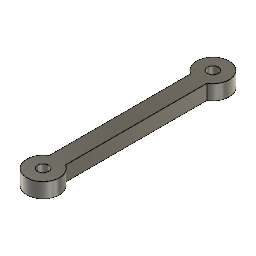
ensamble v16 (Autodesk Fusion 360 archive; units mm, degrees)
design "Eslabon esbelto"
Autodesk Fusion 360 part; units mm, degrees
sketch "Sketch1" plane through (0, 0, 0) normal (0, 1, 0) x (1, 0, 0)
sketch "Sketch2" plane through (0, 0, 0) normal (0, 0, 1) x (1, 0, 0)
  line L0 (-16.2522, 73.2678) -> (-16.2522, 11.1678)
  line L1 (-10.1922, 11.1678) -> (-10.1922, 73.2678)
  circle A0 centre (-13.2222, 73.2678) radius 2
  circle A1 centre (-13.2222, 73.2678) radius 6
  line L2 (-15.6922, 42.2178) -> (-4.6922, 42.2178)
  circle A2 centre (-13.2222, 11.1678) radius 2
  circle A3 centre (-13.2222, 11.1678) radius 6
  dimension "d1" = 6.06
  dimension "d2" = 62.1
  dimension "d3" = 4
  dimension "d4" = 12
  constraint vertical L0
  constraint vertical L1
  constraint concentric A0 A1
  constraint perpendicular L1 L2
  constraint midpoint L1 L2
  constraint symmetric A0 L2 A2
  constraint symmetric A1 L2 A3
  measures "d1" distance of L1.end L0.start
  measures "d2" distance of L1.end L1.start
  measures "d3" diameter of A0
  measures "d4" diameter of A1
extrude "Extrude1" add sketch "Sketch2" along normal blind 5.5
sketch "Sketch3" plane through (0, 0, 5.5) normal (0, 0, 1) x (-1, 0, 0)
  circle A0 centre (13.2222, -11.1678) radius 2
  circle A1 centre (13.2222, -73.2678) radius 2
  arc A2 (16.2522, -16.3465) -> (10.1922, -16.3465) centre (13.2222, -11.1678) ccw
  line L0 (10.1922, -16.3465) -> (10.1922, -68.0891)
  arc A3 (10.1922, -68.0891) -> (16.2522, -68.0891) centre (13.2222, -73.2678) ccw
  line L1 (16.2522, -68.0891) -> (16.2522, -16.3465)
  line L2 (13.2222, -16.3465) -> (21.0096, -16.3465)
  line L3 (21.0096, -16.3465) -> (21.0096, -5.1678)
  line L4 (21.0096, -5.1678) -> (13.2222, -5.1678)
  line L5 (13.2222, -5.1678) -> (13.2222, -16.3465)
  dimension "d10" = 62.1
  dimension "d11" = 68.1
  constraint horizontal L2
  constraint vertical L3
  constraint horizontal L4
  constraint vertical L5
  measures "d10" distance of A0.centre A1.centre
  measures "d11" distance of A1.centre L4

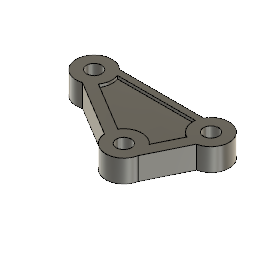
design "triangulo"
Autodesk Fusion 360 part; units mm, degrees
sketch "Sketch1" plane through (0, 0, 0) normal (0, 0, 1) x (1, 0, 0)
  line L0 (3.6773, 16.0313) -> (22.0441, 4.9587)
  line L1 (33.9267, 4.3237) -> (40.3034, 17.2878)
  line L2 (33.9155, 26.0059) -> (6.063, 26.0059)
  circle A0 centre (1.8404, 21.7433) radius 2.5
  circle A1 centre (39.2125, 23.1878) radius 2.5
  circle A2 centre (28.0267, 5.4148) radius 2.5
  circle A3 centre (1.8404, 21.7433) radius 6
  circle A4 centre (39.2125, 23.1878) radius 6
  circle A5 centre (28.0267, 5.4148) radius 6
  line L3 (7.4371, 23.9059) -> (33.2557, 23.9059)
  line L4 (6.7359, 18.2742) -> (22.8989, 8.5302)
  line L5 (32.5192, 9.392) -> (36.639, 17.7677)
  dimension "d6" = 5
  dimension "d7" = 12
  dimension "d8" = 12
  dimension "d9" = 12
  dimension "d10" = 2.1
  dimension "d12" = 3.5
  dimension "d13" = 3.5
  dimension "d23" = 21
  dimension "d25" = 37.4
  dimension "d26" = 30.86
  constraint horizontal L2
  constraint equal A0 A1
  constraint equal A0 A2
  constraint concentric A1 A4
  constraint concentric A2 A5
  constraint concentric A0 A3
  constraint coincident A3 L3.start
  constraint coincident A4 L3.end
  constraint parallel L2 L3
  constraint coincident A3 L4.start
  constraint coincident A5 L4.end
  constraint parallel L0 L4
  constraint coincident A5 L5.start
  constraint coincident A4 L5.end
  constraint parallel L1 L5
  constraint coincident L2.end A3
  constraint coincident L2.start A4
  constraint coincident L1.end A4
  constraint coincident L1.start A5
  constraint coincident L0.start A3
  constraint coincident L0.end A5
  measures "d6" diameter of A0
  measures "d7" diameter of A3
  measures "d8" diameter of A4
  measures "d9" diameter of A5
  measures "d10" distance of L2 L3
  measures "d12" distance of L0 L4
  measures "d13" distance of L1 L5
  measures "d23" distance of A1.centre A2.centre
  measures "d25" distance of A0.centre A1.centre
  measures "d26" distance of A0.centre A2.centre
extrude "Extrude1" add sketch "Sketch1" along normal blind 4 contours L0 A3 A5 L4 | A3 | A5 | L2 A3 A4 L3 | A3 A4 A5 L3 L4 L5 | A4
extrude "Extrude2" add sketch "Sketch1" along normal blind 7 and the other way blind 0.5 contours L0 A3 A5 L4 | A3 | A5 | L2 A3 A4 L3 | L1 A4 A5 L5 | A4
extrude "Extrude4" add 1 faces at (22.1509, 18.7206, 4) along direction (0, 0, 1) blind 2
sketch "Sketch2" plane through (0, 0, 7) normal (0, 0, 1) x (-1, 0, 0)
  circle A0 centre (-39.2125, -23.1878) radius 2.5
  circle A1 centre (-1.8404, -21.7433) radius 2.5
  circle A2 centre (-28.0267, -5.4148) radius 2.5
  line L0 (-3.6773, -16.0313) -> (-22.0441, -4.9587)
  arc A3 (-22.0441, -4.9587) -> (-33.9267, -4.3237) centre (-28.0267, -5.4148) ccw
  line L1 (-33.9267, -4.3237) -> (-40.3034, -17.2878)
  arc A4 (-40.3034, -17.2878) -> (-33.9155, -26.0059) centre (-39.2125, -23.1878) ccw
  line L2 (-33.9155, -26.0059) -> (-6.063, -26.0059)
  arc A5 (-6.063, -26.0059) -> (-3.6773, -16.0313) centre (-1.8404, -21.7433) ccw
sketch "Sketch3" plane through (0, 0, -0.5) normal (0, 0, -1) x (1, 0, 0)
  circle A0 centre (39.2125, -23.1878) radius 2.5
  circle A1 centre (1.8404, -21.7433) radius 2.5
  circle A2 centre (28.0267, -5.4148) radius 2.5
  line L0 (6.7359, -18.2742) -> (22.8989, -8.5302)
  arc A3 (22.8989, -8.5302) -> (32.5192, -9.392) centre (28.0267, -5.4148) ccw
  line L1 (32.5192, -9.392) -> (36.639, -17.7677)
  arc A4 (36.639, -17.7677) -> (33.2557, -23.9059) centre (39.2125, -23.1878) ccw
  line L2 (33.2557, -23.9059) -> (7.4371, -23.9059)
  arc A5 (7.4371, -23.9059) -> (6.7359, -18.2742) centre (1.8404, -21.7433) ccw
  line L3 (22.0441, -4.9587) -> (3.6773, -16.0313)
  arc A6 (3.6773, -16.0313) -> (6.063, -26.0059) centre (1.8404, -21.7433) ccw
  line L4 (6.063, -26.0059) -> (33.9155, -26.0059)
  arc A7 (33.9155, -26.0059) -> (40.3034, -17.2878) centre (39.2125, -23.1878) ccw
  line L5 (40.3034, -17.2878) -> (33.9267, -4.3237)
  arc A8 (33.9267, -4.3237) -> (22.0441, -4.9587) centre (28.0267, -5.4148) ccw
  line L6 (-4.1596, -29.1878) -> (45.2125, -29.1878)
  line L7 (45.2125, -29.1878) -> (45.2125, 0.5852)
  line L8 (45.2125, 0.5852) -> (-4.1596, 0.5852)
  line L9 (-4.1596, 0.5852) -> (-4.1596, -29.1878)
  dimension "d29" = 49.3721
  dimension "d30" = 29.773
  constraint horizontal L6
  constraint vertical L7
  constraint horizontal L8
  constraint vertical L9
  constraint tangent A7 L7
  constraint tangent A6 L9
  constraint tangent A8 L8
  constraint tangent A7 L6
  measures "d29" distance of L7.end L8.end
  measures "d30" distance of L6.start L8.end
equation "d_triang_ext = 16 mm"
equation "d_hueco_m4 = 5 mm"
equation "d6 = d_hueco_m4"
equation "l_borde_tri = 4 mm"
equation "d23 = 16 mm + 5 mm"
equation "d25 = 32.4 mm + 5 mm"
equation "d26 = 25.86 mm + 5 mm"

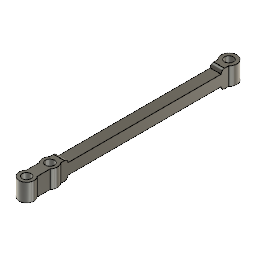
design "Barra marco"
Autodesk Fusion 360 part; units mm, degrees
sketch "Sketch1" plane through (0, 0, 0) normal (0, 0, 1) x (1, 0, 0)
  line L0 (-5, 83.0364) -> (1.2, 83.0364)
  line L1 (1.2, 83.0364) -> (1.2, -30.5636)
  line L2 (1.2, -30.5636) -> (-5, -30.5636)
  line L3 (-5, -30.5636) -> (-5, 83.0364)
  circle A0 centre (-1.9, 83.0364) radius 2.5
  circle A1 centre (-1.9, 83.0364) radius 4.5
  line L4 (-11.3, 26.2364) -> (13.7, 26.2364)
  line L5 (-5, -30.5636) -> (1.2, -30.5636)
  circle A2 centre (-1.9, -30.5636) radius 2.5
  circle A3 centre (-1.9, -30.5636) radius 4.25
  circle A4 centre (-1.9, -17.4636) radius 2.5
  circle A5 centre (-1.9, -17.4636) radius 4.25
  dimension "d1" = 6.2
  dimension "d2" = 113.6
  dimension "d3" = 5
  dimension "d4" = 9
  dimension "d7" = 5
  dimension "d8" = 8.5
  dimension "d9" = 13.1
  dimension "d10" = 8.5
  dimension "d12" = 3.1
  constraint horizontal L0
  constraint vertical L1
  constraint horizontal L2
  constraint vertical L3
  constraint midpoint L0 A0.centre
  constraint concentric A0 A1
  constraint horizontal L4
  constraint midpoint L1 L4
  constraint symmetric L0.start L4 L2.end
  constraint symmetric L0.end L4 L1.end
  constraint symmetric A0 L4 A2
  constraint concentric A4 A5
  measures "d1" distance of L0.start L0.end
  measures "d2" distance of L0.start L2.end
  measures "d3" diameter of A0
  measures "d4" diameter of A1
  measures "d7" diameter of A4
  measures "d8" diameter of A5
  measures "d9" distance of A2.centre A4.centre
  measures "d10" diameter of A3
  measures "d12" distance of L1 A2.centre
extrude "Extrude1" add sketch "Sketch1" along normal blind 6.2 contours L0 L1 L3 A0 A1 | L0 L1 L3 A0 A1 | L1 L3 A1 L4 | L1 L3 L4 A5 | L1 A5 | L1 L3 A5 | L1 L3 A3 A5 | L3 A5 | L1 L2 L3 L5 A2 A3 | L1 L2 L3 L5 A2 A3
sketch "Sketch2" plane through (0, 0, 6.2) normal (0, 0, 1) x (-1, 0, 0)
  circle A0 centre (1.9, 17.4636) radius 2.5
  circle A1 centre (1.9, 30.5636) radius 2.5
  circle A2 centre (1.9, -83.0364) radius 2.5
  arc A3 (5, 27.6563) -> (-1.2, 27.6563) centre (1.9, 30.5636) ccw
  line L0 (-1.2, 27.6563) -> (-1.2, 20.371)
  arc A4 (-1.2, 20.371) -> (-1.2, 14.5563) centre (1.9, 17.4636) ccw
  line L1 (-1.2, 14.5563) -> (-1.2, -79.7745)
  arc A5 (-1.2, -79.7745) -> (5, -79.7745) centre (1.9, -83.0364) ccw
  line L2 (5, -79.7745) -> (5, 14.5563)
  arc A6 (5, 14.5563) -> (5, 20.371) centre (1.9, 17.4636) ccw
  line L3 (5, 20.371) -> (5, 27.6563)
  line L4 (12.6746, 10.4136) -> (-7.3254, 10.4136)
  line L5 (-7.3254, 10.4136) -> (-7.3254, 34.8136)
  line L6 (-7.3254, 34.8136) -> (12.6746, 34.8136)
  line L7 (12.6746, 34.8136) -> (12.6746, 10.4136)
  line L8 (10, -87.5364) -> (-5, -87.5364)
  line L9 (-5, -87.5364) -> (-5, -75.5364)
  line L10 (-5, -75.5364) -> (10, -75.5364)
  line L11 (10, -75.5364) -> (10, -87.5364)
  dimension "d13" = 20
  dimension "d14" = 24.4
  dimension "d15" = 12
  constraint horizontal L4
  constraint vertical L5
  constraint horizontal L6
  constraint vertical L7
  constraint tangent A3 L6
  constraint horizontal L8
  constraint vertical L9
  constraint horizontal L10
  constraint vertical L11
  constraint tangent A5 L8
  measures "d13" distance of L4.start L4.end
  measures "d14" distance of L4.start L6.end
  measures "d15" distance of L8.end L9.end
extrude "Extrude2" add sketch "Sketch2" along normal blind 1.95 contours A3 L0 A4 L1 L2 A6 L3 L4 | L1 A5 L2 L10
ref_plane "WorkPlane1" through (-1.9, 32.5614, 3.1) normal (0, 0, 1) x (1, 0, 0)
fillet "Fillet1" radius 1.95 2 edges at (-1.9, 75.5364, 8.15) (-1.9, -10.4136, 8.15)
mirror "Mirror1" about plane through (-1.9, 32.5614, 3.1) normal (0, 0, 1) of bodies 1 merged
sketch "Sketch3" plane through (0, 0, 0) normal (0, 1, 0) x (1, 0, 0)
  line L0 (-5, 1.95) -> (-5, -8.15)
  line L1 (-6.4, -8.15) -> (2.6, -8.15)
  line L2 (1.2, -8.15) -> (1.2, 1.95)
  line L3 (-6.4, 1.95) -> (2.6, 1.95)
  dimension "d22" = 9
  dimension "d23" = 10.1
  measures "d22" distance of L1.start L1.end
  measures "d23" distance of L1 L3
ref_plane "WorkPlane2" through (0, 0, -15) normal (0, 0, 1) x (1, 0, 0)
ref_plane "WorkPlane3" through (0, 0, 25) normal (0, 0, 1) x (1, 0, 0)
sketch "Sketch4" plane through (0, 0, 25) normal (0, 0, 1) x (1, 0, 0)
  line L0 (-5, 75.5364) -> (-5, -10.4136)
  arc A0 (1.2, 79.7745) -> (-5, 79.7745) centre (-1.9, 83.0364) ccw
  circle A1 centre (-1.9, 83.0364) radius 2.5
  line L1 (-5, 79.7745) -> (-5, 77.4864)
  line L2 (-5, 75.5364) -> (-5, 77.4864)
  line L3 (1.2, 77.4864) -> (1.2, 79.7745)
  line L4 (1.2, 77.4864) -> (1.2, 75.5364)
  line L5 (1.2, -10.4136) -> (1.2, 75.5364)
  line L6 (1.2, -10.4136) -> (1.2, -12.3636)
  line L7 (-5, -12.3636) -> (-5, -10.4136)
  line L8 (-5, -12.3636) -> (-5, -14.5563)
  line L9 (1.2, -14.5563) -> (1.2, -12.3636)
  arc A2 (1.2, -20.371) -> (1.2, -14.5563) centre (-1.9, -17.4636) ccw
  arc A3 (1.2, -20.371) -> (1.2, -14.5563) centre (-1.9, -17.4636) ccw
  circle A4 centre (-1.9, -17.4636) radius 2.5
  arc A5 (-5, -14.5563) -> (-5, -20.371) centre (-1.9, -17.4636) ccw
  line L10 (-5, -12.3636) -> (-5, -14.5563)
  arc A6 (-5, -14.5563) -> (-5, -20.371) centre (-1.9, -17.4636) ccw
  line L11 (-5, -20.371) -> (-5, -27.6563)
  arc A7 (-5, -27.6563) -> (1.2, -27.6563) centre (-1.9, -30.5636) ccw
  line L12 (1.2, -27.6563) -> (1.2, -20.371)
  arc A8 (1.2, -20.371) -> (1.2, -14.5563) centre (-1.9, -17.4636) ccw
  line L13 (1.2, -14.5563) -> (1.2, -12.3636)
  circle A9 centre (-1.9, -30.5636) radius 2.5
  circle A10 centre (-1.9, -17.4636) radius 2.5
equation "d2 = 108.6 mm + 5 mm"
equation "d9 = 8.1 mm + 5 mm"
equation "d12 = d1 / 2"

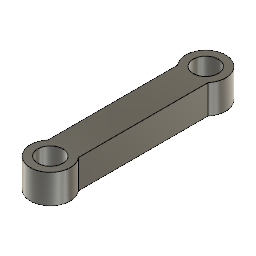
design "Eslabon pequeño"
Autodesk Fusion 360 part; units mm, degrees
sketch "Sketch1" plane through (0, 0, 0) normal (0, 0, 1) x (1, 0, 0)
  line L0 (-5, 25) -> (1.1, 25)
  line L1 (1.1, 25) -> (1.1, -6)
  line L2 (1.1, -6) -> (-5, -6)
  line L3 (-5, -6) -> (-5, 25)
  circle A0 centre (-1.95, 25) radius 2.5
  circle A1 centre (-1.95, 25) radius 4
  line L4 (-10.5, 9.5) -> (0.5, 9.5)
  circle A2 centre (-1.95, -6) radius 4
  circle A3 centre (-1.95, -6) radius 2.5
  line L5 (-5, -6) -> (1.1, -6)
  dimension "d1" = 6.1
  dimension "d2" = 5
  dimension "d3" = 8
  dimension "d6" = 31
  constraint horizontal L0
  constraint vertical L1
  constraint horizontal L2
  constraint vertical L3
  constraint midpoint L0 A0.centre
  constraint concentric A0 A1
  constraint horizontal L4
  constraint midpoint L3 L4
  constraint symmetric L0.start L4 L2.end
  constraint symmetric L0.end L4 L1.end
  constraint symmetric A0 L4 A3
  constraint symmetric A1 L4 A2
  measures "d1" distance of L0.start L0.end
  measures "d2" diameter of A0
  measures "d3" diameter of A1
  measures "d6" distance of A0.centre A2.centre
extrude "Extrude1" add sketch "Sketch1" along normal blind 5.8 contours L0 L1 L3 A0 A1 | L0 L1 L3 A0 A1 | L1 L3 A1 A2 | L1 L2 L3 A2 A3 L5 | L1 L2 L3 A2 A3 L5
sketch "Sketch2" plane through (0, 0, 5.8) normal (0, 0, 1) x (-1, 0, 0)
  circle A0 centre (1.95, -25) radius 2.5
  circle A1 centre (1.95, 6) radius 2.5
  arc A2 (-1.1, -22.412) -> (5, -22.412) centre (1.95, -25) ccw
  line L0 (5, -22.412) -> (5, 3.412)
  arc A3 (5, 3.412) -> (-1.1, 3.412) centre (1.95, 6) ccw
  line L1 (-1.1, 3.412) -> (-1.1, -22.412)
  line L2 (1.95, -29) -> (-2.05, -29)
  line L3 (-2.05, -29) -> (-2.05, 10)
  line L4 (-2.05, 10) -> (1.95, 10)
  line L5 (1.95, 10) -> (1.95, -29)
  line L6 (1.95, -29) -> (5.95, -29)
  line L7 (5.95, -29) -> (5.95, 16.18)
  line L8 (5.95, 16.18) -> (1.95, 16.18)
  line L9 (1.95, 16.18) -> (1.95, -29)
  dimension "d7" = 45.18
  dimension "d8" = 8
  constraint horizontal L2
  constraint vertical L3
  constraint horizontal L4
  constraint vertical L5
  constraint midpoint A2 L2.start
  constraint tangent A2 L3
  constraint tangent A3 L4
  constraint horizontal L6
  constraint vertical L7
  constraint horizontal L8
  constraint vertical L9
  constraint tangent A2 L7
  measures "d7" distance of L6.end L7.end
  measures "d8" distance of L3 L7
equation "d6 = 26 mm + 5 mm"

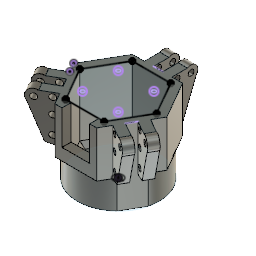
design "Marco"
Autodesk Fusion 360 part; units mm, degrees
sketch "Sketch1" plane through (0, 0, 0) normal (0, 0, 1) x (1, 0, 0)
  line L0 (33.3708, 0) -> (16.6854, 28.9)
  line L1 (16.6854, 28.9) -> (-16.6854, 28.9)
  line L2 (-16.6854, 28.9) -> (-33.3708, 0)
  line L3 (-33.3708, 0) -> (-16.6854, -28.9)
  line L4 (-16.6854, -28.9) -> (16.6854, -28.9)
  line L5 (16.6854, -28.9) -> (33.3708, 0)
  line L6 (40.4145, 1.8) -> (21.7661, 34.1)
  line L7 (21.7661, 34.1) -> (-21.7661, 34.1)
  line L8 (-21.7661, 34.1) -> (-40.4145, 1.8)
  line L9 (-40.4145, 1.8) -> (-18.1022, -36.8462)
  line L10 (-18.1022, -36.8462) -> (18.1022, -36.8462)
  line L11 (18.1022, -36.8462) -> (40.4145, 1.8)
  line L12 (-18.1022, -29.8) -> (-18.1022, -36.8462)
  circle A0 centre (0, 0) radius 35.5
  dimension "d72" = 71
  dimension "d76" = 7
  dimension "d79" = 5.2
  dimension "d80" = 5.2
  dimension "d81" = 5.2
  dimension "d83" = 7
  dimension "d103" = 57.8
  constraint coincident A0.centre origin
  constraint vertical L12
  constraint parallel L2 L8
  measures "d72" diameter of A0
  measures "d76" distance of L0 L6
  measures "d79" distance of L1 L7
  measures "d80" distance of L5 L11
  measures "d81" distance of L3 L9
  measures "d83" distance of L2 L8
  measures "d103" distance of L2 L5
extrude "Extrude1" add sketch "Sketch1" along normal blind 40 contours L6 L7 L11 A0 | L7 L9 L11 A0 | L10 L11 L12 A0 | L7 L8 L9 A0 | L9 L12 A0
sketch "Sketch2" plane through (29.5315, -17.05, 0) normal (0.866025, -0.5, 0) x (0.5, 0.866025, 0)
  line L0 (-22.8586, 0) -> (21.7661, 0)
  line L1 (21.7661, 0) -> (21.7661, 40)
  line L2 (21.7661, 40) -> (-22.8586, 40)
  line L3 (-22.8586, 40) -> (-22.8586, 0)
  line L4 (33.3708, 0) -> (16.6854, 0)
  line L5 (-22.8586, 0) -> (-22.8586, 40)
  line L6 (-22.8586, 40) -> (21.7661, 40)
  line L7 (21.7661, 0) -> (21.7661, 40)
  line L8 (-22.8586, 0) -> (21.7661, 0)
  line L9 (-12.5463, 40) -> (-4.5463, 40)
  line L10 (-4.5463, 40) -> (-4.5463, 0)
  line L11 (-4.5463, 0) -> (-12.5463, 0)
  line L12 (-12.5463, 0) -> (-12.5463, 40)
  line L13 (-0.5463, 40) -> (-0.5463, 34)
  line L14 (11.4537, 40) -> (3.4537, 40)
  line L15 (3.4537, 40) -> (3.4537, 0)
  line L16 (3.4537, 0) -> (11.4537, 0)
  line L17 (11.4537, 0) -> (11.4537, 40)
  dimension "d5" = 8
  dimension "d25" = 8
  constraint horizontal L9
  constraint vertical L10
  constraint horizontal L11
  constraint vertical L12
  constraint coincident L6 L9.start
  constraint midpoint L6 L13.start
  constraint perpendicular L6 L13
  constraint symmetric L9.start L13 L14.start
  constraint symmetric L9.end L13 L14.end
  constraint symmetric L10.end L13 L15.end
  constraint symmetric L11.end L13 L16.end
  measures "d5" distance of L9.start L9.end
  measures "d25" distance of L10 L15
extrude "Extrude2" add sketch "Sketch2" along normal blind 23 contours L0 L2 L6 L8 L9 L10 L11 L12 | L0 L2 L6 L8 L14 L15 L16 L17
sketch "Sketch3" plane through (-6.2731, -10.8654, 0) normal (-0.5, -0.866025, 0) x (0.866025, -0.5, 0)
  line L0 (34.1, 40) -> (34.1, 0)
  line L1 (34.1, 0) -> (57.1, 0)
  line L2 (57.1, 0) -> (57.1, 40)
  line L3 (57.1, 40) -> (34.1, 40)
  line L4 (34.1, 0) -> (43.8551, 2.1993)
  line L5 (43.8551, 2.1993) -> (55.2904, 31.0363)
  circle A0 centre (50.7, 34.9) radius 6
  circle A1 centre (50.7, 34.9) radius 2.5
  line L6 (34.1, 40) -> (53.8607, 40)
  circle A2 centre (38.6, 36.4) radius 2.5
  circle A3 centre (38.6, 23.3) radius 2.5
  circle A4 centre (38.6, 7.9957) radius 2.5
  dimension "d8" = 12
  dimension "d9" = 5
  dimension "d13" = 5
  dimension "d14" = 5
  dimension "d17" = 5
  dimension "d18" = 29.5
  dimension "d19" = 5.1
  dimension "d20" = 16.6
  dimension "d21" = 10
  dimension "d22" = 4.5
  dimension "d23" = 4.5
  dimension "d24" = 4.5
  dimension "d59" = 3.6
  dimension "d60" = 13.1
  constraint coincident L0.end L1.start
  constraint concentric A0 A1
  constraint coincident L5.end A0
  constraint coincident A0 L6.end
  constraint coincident L0.start L3.end
  constraint coincident L3 L6.end
  measures "d8" diameter of A0
  measures "d9" diameter of A1
  measures "d13" diameter of A2
  measures "d14" diameter of A3
  measures "d17" diameter of A4
  measures "d18" distance of A0.centre A4.centre
  measures "d19" distance of A0.centre L6
  measures "d20" distance of L0 A0.centre
  measures "d21" distance of L0.end L4.end
  measures "d22" distance of L0 A4.centre
  measures "d23" distance of L0 A3.centre
  measures "d24" distance of L0 A2.centre
  measures "d59" distance of L6 A2.centre
  measures "d60" distance of A2.centre A3.centre
extrude "Extrude4" add sketch "Sketch3" against normal blind 8 contours L3 A0 L6 picked at (50.7, 40.3)
extrude "Extrude5" add sketch "Sketch3" against normal blind 8 from surface at -16 contours L3 A0 L6 picked at (50.7, 40.3)
extrude "Extrude6" cut sketch "Sketch3" against normal blind 47 contours L1 L2 L3 L4 L5 A0
extrude "Extrude7" cut sketch "Sketch3" against normal blind 40 contours A1
extrude "Extrude8" cut sketch "Sketch3" against normal blind 50 contours A4
extrude "Extrude10" add sketch "Sketch1" along normal blind 40 contours L7 L9 L11 A0
extrude "Extrude11" add sketch "Sketch1" against normal blind 25 contours L11 A0 | L7 L9 L11 A0 | L7 A0 | L9 A0
extrude "Extrude3" cut sketch "Sketch3" against normal blind 139 contours L1 L2 L3 L4 L5 A0 | A1 | A2 | A3
pattern_circular "C-Pattern1" count 3 over 360 about axis through (0, 0, 1.75) along (0, 0, 1) of "Extrude2", "Extrude4", "Extrude5", "Extrude8", "Extrude3"
sketch "Sketch4" plane through (0, 0, -25) normal (0, 0, -1) x (1, 0, 0)
  circle A0 centre (0, 0) radius 35.5
  circle A1 centre (0, 0) radius 43.3013
  line L0 (16.6854, 28.9) -> (33.3708, 0)
  line L1 (33.3708, 0) -> (16.6854, -28.9)
  line L2 (16.6854, -28.9) -> (-16.6854, -28.9)
  line L3 (-16.6854, -28.9) -> (-33.3708, 0)
  line L4 (-33.3708, 0) -> (-16.6854, 28.9)
  line L5 (-16.6854, 28.9) -> (16.6854, 28.9)
  constraint concentric A0 A1
extrude "Extrude12" add sketch "Sketch4" against normal blind 7.1 contours L0 L1 L2 L3 L4 L5
sketch "Sketch5" plane through (0, 0, -25) normal (0, 0, -1) x (1, 0, 0)
  circle A0 centre (0, 0) radius 35.5
  circle A1 centre (0, 0) radius 4
  dimension "d49" = 8
  constraint coincident A0.centre A1.centre
  measures "d49" diameter of A1
extrude "Extrude13" cut sketch "Sketch5" against normal blind 110 contours A1
sketch "Sketch6" plane through (0, -36.8462, 0) normal (0, -1, 0) x (1, 0, 0)
  line L0 (-18.1022, 0) -> (18.1022, 0)
  line L1 (18.1022, 0) -> (18.1022, 40)
  line L2 (18.1022, 40) -> (-18.1022, 40)
  line L3 (-18.1022, 40) -> (-18.1022, 0)
  line L4 (-12, 40) -> (12, 40)
  line L5 (12, 40) -> (12, 10.3)
  line L6 (12, 10.3) -> (-12, 10.3)
  line L7 (-12, 10.3) -> (-12, 40)
  line L8 (-18.1022, 40) -> (18.1022, 40)
  line L9 (-18.1022, 40) -> (18.1022, 40)
  line L10 (18.1022, 40) -> (18.1022, 0)
  line L11 (18.1022, 0) -> (-18.1022, 0)
  line L12 (-18.1022, 0) -> (-18.1022, 40)
  dimension "d52" = 24
  dimension "d53" = 29.7
  dimension "d55" = 36.2043
  dimension "d56" = 6.1022
  constraint horizontal L4
  constraint vertical L5
  constraint horizontal L6
  constraint vertical L7
  constraint coincident L2 L4.start
  constraint horizontal L9
  constraint vertical L10
  constraint horizontal L11
  constraint vertical L12
  constraint coincident L0.end L1.start
  constraint coincident L2.end L3.start
  measures "d52" distance of L4.start L4.end
  measures "d53" distance of L4.start L6.end
  measures "d55" distance of L10 L12
  measures "d56" distance of L5 L10
extrude "Extrude14" cut sketch "Sketch6" against normal blind 20 contours L2 L4 L5 L6 L7 L8 L9
sketch "Sketch7" plane through (0, 0, -17.9) normal (0, 0, 1) x (-1, 0, 0)
  circle A0 centre (0, 0) radius 4
  line L0 (-16.6854, 28.9) -> (-33.3708, 0)
  line L1 (33.3708, 0) -> (16.6854, 28.9)
  circle A1 centre (0, 0) radius 4
  circle A2 centre (0, 0) radius 10
  line L2 (16.6854, 28.9) -> (-16.6854, 28.9)
  line L3 (-33.3708, 0) -> (-16.6854, -28.9)
  line L4 (-16.6854, -28.9) -> (16.6854, -28.9)
  line L5 (16.6854, -28.9) -> (33.3708, 0)
  line L6 (15.5, -15.5) -> (-15.5, -15.5)
  line L7 (-15.5, -15.5) -> (-15.5, 15.5)
  line L8 (-15.5, 15.5) -> (15.5, 15.5)
  line L9 (15.5, 15.5) -> (15.5, -15.5)
  circle A3 centre (15.5, -15.5) radius 1.5
  circle A4 centre (-15.5, -15.5) radius 1.5
  circle A5 centre (15.5, 15.5) radius 1.5
  circle A6 centre (-15.5, 15.5) radius 1.5
  line L10 (-17.15, 21.15) -> (17.15, 21.15)
  line L11 (21.15, 17.15) -> (21.15, -17.15)
  line L12 (17.15, -21.15) -> (-17.15, -21.15)
  line L13 (-21.15, -17.15) -> (-21.15, 17.15)
  arc A7 (-17.15, 21.15) -> (-21.15, 17.15) centre (-17.15, 17.15) ccw
  arc A8 (21.15, 17.15) -> (17.15, 21.15) centre (17.15, 17.15) ccw
  arc A9 (17.15, -21.15) -> (21.15, -17.15) centre (17.15, -17.15) ccw
  arc A10 (-21.15, -17.15) -> (-17.15, -21.15) centre (-17.15, -17.15) ccw
  point P0 (-21.15, 21.15)
  point P1 (21.15, 21.15)
  point P2 (-21.15, -21.15)
  dimension "d61" = 8
  dimension "d62" = 20
  dimension "d85" = 31
  dimension "d86" = 31
  dimension "d87" = 15.5
  dimension "d88" = 15.5
  dimension "d89" = 3
  dimension "d90" = 3
  dimension "d91" = 3
  dimension "d92" = 3
  dimension "d95" = 42.3
  dimension "d96" = 42.3
  dimension "d97" = 21.15
  dimension "d98" = 21.15
  dimension "d99" = 4
  dimension "d100" = 4
  dimension "d101" = 4
  dimension "d102" = 4
  constraint coincident A0.centre A1.centre
  constraint coincident L6.start L9.end
  constraint coincident L6.end L7.start
  constraint coincident L8.end L9.start
  constraint coincident L7.end L8.start
  constraint perpendicular L10 L13
  constraint perpendicular L10 L11
  constraint perpendicular L11 L12
  constraint perpendicular L8 L9
  constraint perpendicular L6 L9
  constraint perpendicular L6 L7
  constraint parallel L8 L10
  constraint coincident P0 L10
  constraint coincident P0 L13
  constraint tangent L10 A7
  constraint tangent L13 A7
  constraint coincident P1 L10
  constraint coincident P1 L11
  constraint tangent L10 A8
  constraint tangent L11 A8
  constraint tangent L11 A9
  constraint tangent L12 A9
  constraint coincident P2 L13
  constraint coincident P2 L12
  constraint tangent L13 A10
  constraint tangent L12 A10
  measures "d61" diameter of A1
  measures "d62" diameter of A2
  measures "d85" distance of L6.start L6.end
  measures "d86" distance of L6.start L8.end
  measures "d87" distance of A0.centre L7
  measures "d88" distance of A0.centre L6
  measures "d89" diameter of A3
  measures "d90" diameter of A4
  measures "d91" diameter of A5
  measures "d92" diameter of A6
  measures "d95" distance of P0 P1
  measures "d96" distance of P0 P2
  measures "d97" distance of A0.centre L11
  measures "d98" distance of A0.centre L12
  measures "d99" radius of A7
  measures "d100" radius of A8
  measures "d101" radius of A9
  measures "d102" radius of A10
extrude "Extrude15" add sketch "Sketch7" along normal blind 9.9 contours A2
sketch "Sketch8" plane through (0, 0, -25) normal (0, 0, -1) x (1, 0, 0)
  circle A0 centre (0, 0) radius 4
  circle A1 centre (0, 0) radius 35.5
  circle A2 centre (0, 0) radius 2.35
  circle A3 centre (0, 0) radius 4
  dimension "d65" = 4.7
  dimension "d66" = 8
  constraint coincident A0.centre A1.centre
  constraint concentric A2 A3
  measures "d65" diameter of A2
  measures "d66" diameter of A3
sketch "Sketch9" plane through (0, 0, -8) normal (0, 0, 1) x (-1, 0, 0)
  circle A0 centre (0, 0) radius 4
  circle A1 centre (0, 0) radius 10
  circle A2 centre (0, 0) radius 2.35
  circle A3 centre (0, 0) radius 4
  dimension "d67" = 4.7
  constraint coincident A0.centre A1.centre
  measures "d67" diameter of A2
extrude "Extrude16" add sketch "Sketch9" against normal up to surface (6.9 mm away) from surface at -10.1 contours A0 A3
extrude "Extrude17" cut sketch "Sketch1" against normal blind 35 contours L11 A0 | L7 A0 | L9 A0
chamfer "Chamfer2" distance 4 angle 45 6 edges at (25.0281, -14.45, -17.9) (0, -28.9, -17.9) (-25.0281, 14.45, -17.9) (0, 28.9, -17.9) (25.0281, 14.45, -17.9) (-25.0281, -14.45, -17.9)
sketch "Sketch10" plane through (0, 0, 40) normal (0, 0, 1) x (-1, 0, 0)
  line L0 (12, 36.8462) -> (12, 28.9)
  line L1 (12, 28.9) -> (16.6854, 28.9)
  line L2 (16.6854, 28.9) -> (33.3708, 0)
  line L3 (33.3708, 0) -> (16.6854, -28.9)
  line L4 (16.6854, -28.9) -> (-16.6854, -28.9)
  line L5 (-16.6854, -28.9) -> (-33.3708, 0)
  line L6 (-33.3708, 0) -> (-16.6854, 28.9)
  line L7 (-16.6854, 28.9) -> (-12, 28.9)
  line L8 (-12, 28.9) -> (-12, 36.8462)
  line L9 (-12, 36.8462) -> (-18.1022, 36.8462)
  line L10 (-18.1022, 36.8462) -> (-23.2583, 27.9154)
  line L11 (-23.2583, 27.9154) -> (-34.8971, 34.635)
  line L12 (-34.8971, 34.635) -> (-38.8971, 27.7068)
  line L13 (-38.8971, 27.7068) -> (-27.2583, 20.9872)
  line L14 (-31.2583, 14.059) -> (-42.8971, 20.7786)
  line L15 (-42.8971, 20.7786) -> (-46.8971, 13.8504)
  line L16 (-46.8971, 13.8504) -> (-35.2583, 7.1308)
  line L17 (-35.2583, 7.1308) -> (-40.4145, -1.8)
  line L18 (-40.4145, -1.8) -> (-21.7661, -34.1)
  line L19 (-21.7661, -34.1) -> (-12.5463, -34.1)
  line L20 (-12.5463, -34.1) -> (-12.5463, -47.5393)
  line L21 (-12.5463, -47.5393) -> (-4.5463, -47.5393)
  line L22 (-4.5463, -47.5393) -> (-4.5463, -34.1)
  line L23 (3.4537, -34.1) -> (3.4537, -47.5393)
  line L24 (3.4537, -47.5393) -> (11.4537, -47.5393)
  line L25 (11.4537, -47.5393) -> (11.4537, -34.1)
  line L26 (11.4537, -34.1) -> (21.7661, -34.1)
  line L27 (21.7661, -34.1) -> (40.4145, -1.8)
  line L28 (31.8046, 13.1128) -> (27.8046, 20.041)
  line L29 (35.8046, 6.1846) -> (47.4434, 12.9043)
  line L30 (47.4434, 12.9043) -> (43.4434, 19.8325)
  line L31 (43.4434, 19.8325) -> (31.8046, 13.1128)
  line L32 (27.8046, 20.041) -> (39.4434, 26.7607)
  line L33 (39.4434, 26.7607) -> (35.4434, 33.6889)
  line L34 (35.4434, 33.6889) -> (23.8046, 26.9692)
  line L35 (23.8046, 26.9692) -> (18.1022, 36.8462)
  line L36 (18.1022, 36.8462) -> (12, 36.8462)
  line L37 (33.3708, 0) -> (16.6854, -28.9)
  line L38 (16.6854, -28.9) -> (-16.6854, -28.9)
  line L39 (-16.6854, -28.9) -> (-33.3708, 0)
  line L40 (-33.3708, 0) -> (-16.6854, 28.9)
  line L41 (-16.6854, 28.9) -> (16.6854, 28.9)
  line L42 (16.6854, 28.9) -> (33.3708, 0)
  circle A0 centre (15.5, -15.5) radius 1.5
  circle A1 centre (15.5, 15.5) radius 1.5
  circle A2 centre (-15.5, 15.5) radius 1.5
  circle A3 centre (-15.5, -15.5) radius 1.5
  line L43 (40.4145, -1.8) -> (35.8046, 6.1846)
  line L44 (-27.2583, 20.9872) -> (-31.2583, 14.059)
  line L45 (-4.5463, -34.1) -> (3.4537, -34.1)
  constraint coincident L2.end L3.start
  constraint coincident L3.end L4.start
  constraint coincident L4.end L5.start
  constraint coincident L5.end L6.start
  constraint coincident L6.end L7.start
  constraint coincident L1.end L2.start
equation "d22 = 2 mm + 2.5 mm"
equation "d53 = 40 mm - 10.3 mm"
equation "d56 = d55 / 2 - 12 mm"
equation "d59 = 1.1 mm + 2.5 mm"
equation "d60 = 8.1 mm + 5 mm"
equation "d79 = d81"
equation "d80 = d79"
equation "d87 = ( 31 / 2 ) * 1 mm"
equation "d88 = ( 31 / 2 ) * 1 mm"
equation "d97 = ( 42.3 / 2 ) * 1 mm"
equation "d98 = ( 42.3 / 2 ) * 1 mm"
